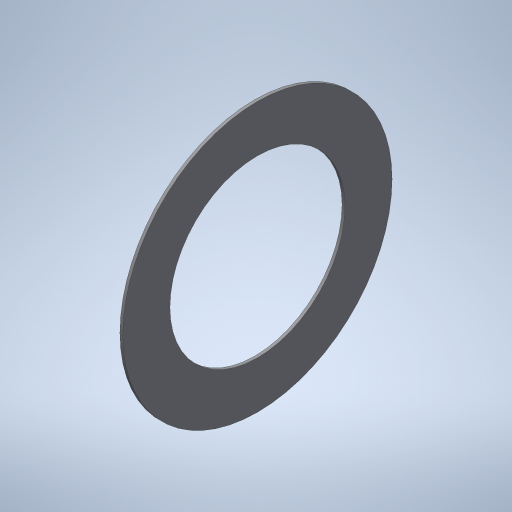
# Autodesk Inventor part: RF-2210X2HH_shield
Saved by Autodesk Inventor 2024.3 (Build 283343010, 343A)
## iProperties
Created: 2019-07-25
Part Number: RF-2210X2HH_shield
Material: 一般
Catalog Web Link: www.cadenas.de
Description: Radial Flanged Ball Bearings (RF-Series/LF series) Metric ST shield-Radial Flanged Ball Bearings (RF-Series/LF series) Metric Shielded Type
Vendor: NMB
Document SubType Name: Modeling
Designer: psadmin
Manufacturer: NMB
Mass: 0.0330317 g
Surface Area: 3.50097 cm^2
Volume: 0.0330317 cm^3
Density: 1 g/cm^3
Appearance: PSOLRGB-192-192-192
Category: PARTsolutions
Company: NMB
PSOL_IDENT_0: {$CADENAS_DATA\23d-libs\nmb\pbbp\radial_flanged_ball_bearings\rfbb_rflfs_m\rflf_shielded_shield.prj}
PSOL_IDENT_1: ,239 {VTYP=3D},{NB=RF-2210X2HH_shield},{LINA=RF-2210X2HH_shield},{NN=Radial Flanged Ball Bearings (R
PSOL_IDENT_2: F-Series/LF series) Metric ST shield},{DATE=11.11.2013 05:13:45},{GEOMDATE=24.10.2013 09:56:00},{VER
PSOL_IDENT_3: SION=},{LINEID=1560},{WBVAR=},{WBNUMERIC=}  {NB=RF-2210X2HH_shield},{LINA=RF-2210X2HH_shield},{KT=DU
PSOL_IDENT_4: MMY},{IDNR=},{PN=RF-2210X2HH},{SHLD=shielded},{FLANG=flanged},{SD=10.000},{D=22.000},{B=6.000},{SR=0
PSOL_IDENT_5: .30},{BCZ=9},{DW=3.1750},{LI=12.40},{LO=19.08},{D1=25.000},{C1=1.50},{D2=0.0},{C2=0.00},{COR=1273},{
PSOL_IDENT_6: CR=1065},{PCD=16.000},{U=19.175},{W=12.825},{Y=1.588},{Z=1.588},{AA=18.858},{AC=1.20},{AD=0.000},{AF=
PSOL_IDENT_7: 0.00},{AQ=0.20},{AH=19.28},{AI=12.60},{AJ=0.40}
NN: Radial Flanged Ball Bearings (RF-Series/LF series) Metric ST shield
NT: Radial Flanged Ball Bearings (RF-Series/LF series) Metric Shielded Type
NB: RF-2210X2HH_shield
NBSYN: $PN._shield
LINA: RF-2210X2HH_shield
PN: RF-2210X2HH
SHLD: shielded
FLANG: flanged
SD: 10
D: 22
B: 6
SR: 0.3
BCZ: 9
DW: 3.175
LI: 12.4
LO: 19.08
D1: 25
C1: 1.5
D2: 0
C2: 0
COR: 1273
CR: 1065
PCD: 16
U: 19.175
W: 12.825
Y: 1.588
Z: 1.588
AA: 18.858
AC: 1.2
AD: 0
AF: 0
AQ: 0.2
AH: 19.28
AI: 12.6
AJ: 0.4
SUPPLIER: NMB
ARTICLENO: RF-2210X2HH_shield
BOMINFO: RF-2210X2HH_shield
CREATOR: CADENAS GmbH
Title: RF-2210X2HH_shield
Author: Cadenas PARTsolutions
Comments: Radial Flanged Ball Bearings (RF-Series/LF series) Metric Shielded Type
Autodesk Inventor part; units mm, degrees
sketch "Sketch_1" plane through (0, 0, 0) normal (0, 0, 1) x (1, 0, 0)
  line L0 (0.2, 0) -> (0, 0)
  line L1 (0, 9.54) -> (0, 6.2)
  line L2 (0, 6.2) -> (0.2, 6.2)
  line L3 (0.2, 6.2) -> (0.2, 9.54)
  line L4 (0.2, 9.54) -> (0, 9.54)
  constraints: 10 end point
revolve "Revolution1" add sketch "Sketch_1" angle 360 about axis through (0.2, 0, 0) along (1, 0, 0)
ref_plane "1_XY" through (0, 0, 0) normal (1, 0, 0) x (0, 0, -1)
ref_plane "1_YZ" through (0, 0, 0) normal (0, 0, -1) x (0, 1, 0)
ref_plane "1_ZX" through (0, 0, 0) normal (0, 1, 0) x (1, 0, 0)
body "Solid1"
